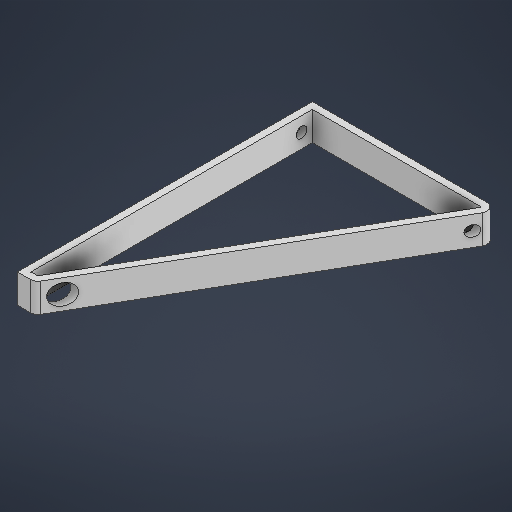
# Autodesk Inventor part: FL-LapTimer-Foot
Saved by Autodesk Inventor 2026 (Build 300175000, 175)
## iProperties
Created: 2026-03-25
Part Number: FL-LapTimer-Foot
Material: Všeobecné
Document SubType Name: Modeling
Designer: vadim
Density: 1 g/cm^3
Appearance: Výchozí
Author: vadim
Autodesk Inventor part; units mm, degrees
ref_plane "YZ Plane" through (0, 0, 0) normal (1, 0, 0) x (0, 1, 0)
ref_plane "XZ Plane" through (0, 0, 0) normal (0, 1, 0) x (-1, 0, 0)
ref_plane "XY Plane" through (0, 0, 0) normal (0, 0, 1) x (1, 0, 0)
sketch "Náčrt1" plane through (0, 0, 0) normal (0, 1, 0) x (-1, 0, 0)
  line L0 (0, 0) -> (0, 83)
  line L1 (0, 83) -> (-2, 83)
  line L2 (-2, 83) -> (-49.9201, 0)
  line L3 (-49.9201, 0) -> (0, 0)
  line L4 (2, 85) -> (2, -2)
  line L5 (2, -2) -> (-53.3842, -2)
  line L6 (-53.3842, -2) -> (-3.1547, 85)
  line L7 (-3.1547, 85) -> (2, 85)
  dimension "d0" = 30
  dimension "d1" = 2
  dimension "d2" = 83
  dimension "d3" = 49.9201
  dimension "d4" = 2
  constraints: 16 end point, 2 parallel, 2 perpendicular, 1 vertical, 3 other
  measures "d0" angle of L0 L2
  measures "d1" distance of L0.end L1.end
  measures "d2" distance of L0.start L0.end
  measures "d3" distance of L2.end L0.start
  measures "d4" distance between parallel lines of L0 L4
extrude "Vysunutí1" add sketch "Náčrt1" along normal blind 8.5
sketch "Náčrt2" plane through (-2, 0, -2) normal (-1, 0, 0) x (0, 0, 1)
  line L0 (0, 0) -> (87, 0) projected
  line L1 (87, 0) -> (87, 8.5) projected
  line L2 (0, 8.5) -> (87, 8.5) projected
  line L3 (0, 0) -> (0, 8.5) projected
  line L4 (0, 4.25) -> (87, 4.25) construction
  circle A0 centre (5.2, 4.25) radius 1.5
  circle A1 centre (81.8, 4.25) radius 1.5
  line L5 (43.5, 8.5) -> (43.5, 0) construction
  circle A2 centre (5.2, 4.25) radius 3
  circle A3 centre (81.8, 4.25) radius 3
  point P0 (2, 0)
  dimension "d10" = 3
  dimension "d11" = 38.3
  dimension "d12" = 76.6
  dimension "d13" = 6
  constraints: 4 centre point, 4 end point, 4 midpoint, 2 point on line, 1 coincident, 1 symmetric about line, 2 other
  measures "d10" diameter of A0
  measures "d11" distance from line of A0.centre L5
  measures "d12" distance of A0.centre A1.centre
  measures "d13" diameter of A2
hole "Díra1" at (-2, 4.25, 79.8) at (-2, 4.25, 3.2) direction (1, 0, 0) diameter 3.2 end through all
extrude "Vysunutí2" cut sketch "Náčrt2" against normal blind 11.25 contours A3
extrude "Vysunutí3" add sketch "Náčrt2" against normal up to surface (2 mm away) contours A3
fillet "Zaoblení1" radius 2.25 2 edges at (53.3842, 4.25, -2) (3.1547, 4.25, 85)
fillet "Zaoblení1" radius 0.25 2 edges at (49.9201, 4.25, 0) (2, 4.25, 83)
